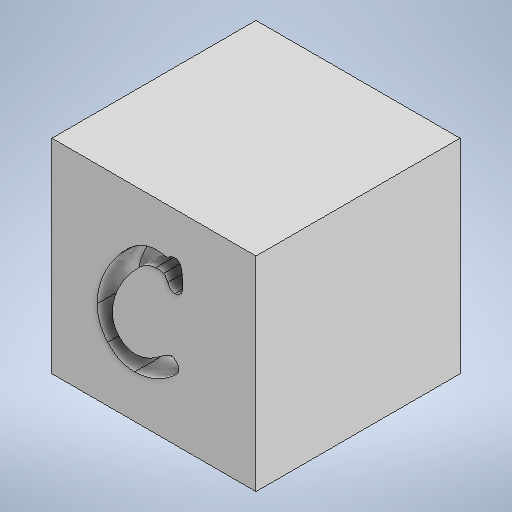
# Autodesk Inventor part: Cytosine
Saved by Autodesk Inventor 2025 (Build 290162000, 162)
## iProperties
Created: 2024-08-12
Part Number: Cytosine
Material: Generic
Document SubType Name: Modeling
Designer: kellst1
Density: 1 g/cm^3
Appearance: Default
Author: kellst1
Autodesk Inventor part; units mm, degrees
ref_plane "YZ Plane" through (0, 0, 0) normal (1, 0, 0) x (0, 1, 0)
ref_plane "XZ Plane" through (0, 0, 0) normal (0, 1, 0) x (-1, 0, 0)
ref_plane "XY Plane" through (0, 0, 0) normal (0, 0, 1) x (1, 0, 0)
sketch "Sketch1" plane through (0, 0, 0) normal (1, 0, 0) x (0, 1, 0)
  line L0 (0, 0) -> (10, 0)
  line L1 (10, 0) -> (10, -10)
  line L2 (10, -10) -> (0, -10)
  line L3 (0, -10) -> (0, 0)
  dimension "d0" = 10
  dimension "d1" = 10
  constraints: 8 end point, 2 parallel, 1 horizontal, 1 perpendicular
  measures "d0" distance of L1.end L2.end
  measures "d1" distance of L0.end L1.end
extrude "Extrusion1" add sketch "Sketch1" along normal blind 10
sketch "Sketch3" plane through (0, 0, 0) normal (-1, 0, 0) x (0, 0, 1)
  circle A0 centre (-5, 5) radius 1.5
  point P0 (0, 0)
  constraints: 1 centre point
extrude "Extrusion3" cut sketch "Sketch3" against normal blind 5
sketch "Sketch4" plane through (0, 0, 0) normal (0, 0, 1) x (1, 0, 0)
  line L0 (1.8731, 7.9408) -> (4.4271, 7.9408) construction
  line L1 (4.4271, 7.9408) -> (4.4271, 4.8928) construction
  line L2 (4.4271, 4.8928) -> (1.8731, 4.8928) construction
  line L3 (1.8731, 4.8928) -> (1.8731, 7.9408) construction
  spline S0 degree 2 poles (6.0379, 6.4263) (5.7961, 6.4263) (5.6751, 6.7102) knots 0 0 0 1 1 1
  spline S1 degree 2 poles (5.6751, 6.7102) (5.5699, 6.9521) (5.4805, 7.0047) knots 0 0 0 1 1 1
  spline S2 degree 2 poles (5.4805, 7.0047) (5.4017, 7.0468) (5.0861, 7.0468) knots 0 0 0 1 1 1
  spline S3 degree 2 poles (5.0861, 7.0468) (4.5392, 7.0468) (3.8714, 6.2107) knots 0 0 0 1 1 1
  spline S4 degree 2 poles (3.8714, 6.2107) (2.9669, 5.0853) (2.9669, 4.0809) knots 0 0 0 1 1 1
  spline S5 degree 2 poles (2.9669, 4.0809) (2.9669, 3.5919) (3.2824, 3.2448) knots 0 0 0 1 1 1
  spline S6 degree 2 poles (3.2824, 3.2448) (3.6032, 2.882) (4.0554, 2.882) knots 0 0 0 1 1 1
  spline S7 degree 2 poles (4.0554, 2.882) (4.4446, 2.882) (4.8337, 3.0818) knots 0 0 0 1 1 1
  spline S8 degree 2 poles (4.8337, 3.0818) (5.0546, 3.1975) (5.5068, 3.5288) knots 0 0 0 1 1 1
  spline S9 degree 2 poles (5.5068, 3.5288) (5.7224, 3.6865) (5.8329, 3.6865) knots 0 0 0 1 1 1
  spline S10 degree 2 poles (5.8329, 3.6865) (5.9906, 3.6865) (6.2115, 3.4394) (6.2115, 3.2921) knots 0 0 0 1 2 2 2
  spline S11 degree 2 poles (6.2115, 3.2921) (6.2115, 3.1186) (6.0695, 2.9924) knots 0 0 0 1 1 1
  spline S12 degree 2 poles (6.0695, 2.9924) (5.0704, 2.1089) (4.0554, 2.1089) knots 0 0 0 1 1 1
  spline S13 degree 2 poles (4.0554, 2.1089) (3.2719, 2.1089) (2.7355, 2.7084) knots 0 0 0 1 1 1
  spline S14 degree 2 poles (2.7355, 2.7084) (2.2149, 3.2869) (2.2149, 4.0809) knots 0 0 0 1 1 1
  spline S15 degree 2 poles (2.2149, 4.0809) (2.2149, 5.3588) (3.2877, 6.6997) knots 0 0 0 1 1 1
  spline S16 degree 2 poles (3.2877, 6.6997) (4.1817, 7.8198) (5.0861, 7.8198) knots 0 0 0 1 1 1
  spline S17 degree 2 poles (5.0861, 7.8198) (5.2702, 7.8198) (5.5647, 7.7883) (5.6804, 7.7462) knots 0 0 0 1 2 2 2
  spline S18 degree 2 poles (5.6804, 7.7462) (5.8118, 7.9408) (6.0222, 7.9408) knots 0 0 0 1 1 1
  spline S19 degree 2 poles (6.0222, 7.9408) (6.2851, 7.9408) (6.3535, 7.5989) knots 0 0 0 1 1 1
  spline S20 degree 2 poles (6.3535, 7.5989) (6.4113, 7.2887) (6.4113, 6.847) knots 0 0 0 1 1 1
  spline S21 degree 2 poles (6.4113, 6.847) (6.4113, 6.6892) (6.3272, 6.5735) knots 0 0 0 1 1 1
  spline S22 degree 2 poles (6.3272, 6.5735) (6.2273, 6.4263) (6.0379, 6.4263) knots 0 0 0 1 1 1
  point P0 (0, 0)
  constraints: 2 other
extrude "Extrusion4" cut sketch "Sketch4" against normal blind 2
body "Solid1"
